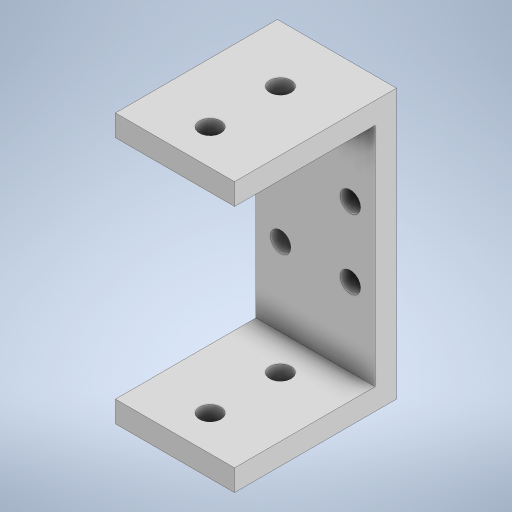
# Autodesk Inventor part: AcopleActuadorCarro
Saved by Autodesk Inventor 2023 (Build 270158000, 158)
## iProperties
Created: 2023-04-08
Part Number: AcopleActuadorCarro
Material: Generic
Document SubType Name: Modeling
Designer: Lenovo
Density: 1 g/cm^3
Appearance: Default
Author: Lenovo
Autodesk Inventor part; units mm, degrees
ref_plane "YZ Plane" through (0, 0, 0) normal (1, 0, 0) x (0, 1, 0)
ref_plane "XZ Plane" through (0, 0, 0) normal (0, 1, 0) x (-1, 0, 0)
ref_plane "XY Plane" through (0, 0, 0) normal (0, 0, 1) x (1, 0, 0)
sketch "Sketch1" plane through (0, 0, 0) normal (0, 0, 1) x (1, 0, 0)
  line L0 (-6, 110.6647) -> (-6, 110.2647)
  arc A0 (-6, 110.2647) -> (-5.6, 109.8647) centre (-5.6, 110.2647) ccw
  line L1 (-5.6, 109.8647) -> (-4.9, 109.8647)
  arc A1 (-4.9, 109.8647) -> (-4.7, 110.0647) centre (-4.9, 110.0647) ccw
  line L2 (-4.7, 110.0647) -> (-4.7, 110.3147)
  arc A2 (-4.5, 110.5147) -> (-4.7, 110.3147) centre (-4.5, 110.3147) ccw
  line L3 (-4.5, 110.5147) -> (-1.8, 110.5147)
  arc A3 (-1.4, 110.1147) -> (-1.8, 110.5147) centre (-1.8, 110.1147) ccw
  line L4 (-1.4, 110.1147) -> (-1.4, 104.4147)
  line L5 (-1.8, 104.0147) -> (-4.5, 104.0147)
  arc A4 (-1.8, 104.0147) -> (-1.4, 104.4147) centre (-1.8, 104.4147) ccw
  arc A5 (-4.7, 104.2147) -> (-4.5, 104.0147) centre (-4.5, 104.2147) ccw
  line L6 (-4.7, 104.2147) -> (-4.7, 104.4647)
  arc A6 (-4.7, 104.4647) -> (-4.9, 104.6647) centre (-4.9, 104.4647) ccw
  line L7 (-4.9, 104.6647) -> (-5.6, 104.6647)
  arc A7 (-5.6, 104.6647) -> (-6, 104.2647) centre (-5.6, 104.2647) ccw
  line L8 (-6, 104.2647) -> (-6, 103.6647)
  line L9 (-6.5, 116.6647) -> (-6.5, 110.6647)
  line L10 (-6.5, 110.6647) -> (-2.5, 110.6647)
  line L11 (-1.05, 103.6647) -> (-6.5, 103.6647)
  line L12 (-6.5, 103.6647) -> (-6.5, 97.1647)
  line L13 (-6.5, 97.1647) -> (-1.05, 97.1647)
  line L14 (-6, 97.1647) -> (-6, 96.5647)
  arc A8 (-6, 96.5647) -> (-5.6, 96.1647) centre (-5.6, 96.5647) ccw
  line L15 (-5.6, 96.1647) -> (-4.9, 96.1647)
  arc A9 (-4.9, 96.1647) -> (-4.7, 96.3647) centre (-4.9, 96.3647) ccw
  arc A10 (-4.5, 96.8147) -> (-4.7, 96.6147) centre (-4.5, 96.6147) ccw
  line L16 (-4.7, 96.3647) -> (-4.7, 96.6147)
  line L17 (-4.5, 96.8147) -> (-1.8, 96.8147)
  arc A11 (-1.4, 96.4147) -> (-1.8, 96.8147) centre (-1.8, 96.4147) ccw
  line L18 (-1.4, 96.4147) -> (-1.4, 90.7147)
  arc A12 (-1.8, 90.3147) -> (-1.4, 90.7147) centre (-1.8, 90.7147) ccw
  line L19 (-1.8, 90.3147) -> (-4.5, 90.3147)
  arc A13 (-4.7, 90.5147) -> (-4.5, 90.3147) centre (-4.5, 90.5147) ccw
  line L20 (-4.7, 90.5147) -> (-4.7, 90.7647)
  arc A14 (-4.7, 90.7647) -> (-4.9, 90.9647) centre (-4.9, 90.7647) ccw
  line L21 (-4.9, 90.9647) -> (-5.6, 90.9647)
  arc A15 (-5.6, 90.9647) -> (-6, 90.5647) centre (-5.6, 90.5647) ccw
  line L22 (-6, 90.5647) -> (-6, 90.1647)
  line L23 (-2.5, 90.1647) -> (-6.5, 90.1647)
  line L24 (-6.5, 90.1647) -> (-6.5, 84.1647)
  line L25 (32.5, 123.1647) -> (0, 123.1647)
  circle A16 centre (0, 116.6647) radius 4.75
  circle A17 centre (32.5, 116.6647) radius 4.75
  circle A18 centre (0, 84.1647) radius 4.75
  circle A19 centre (32.5, 84.1647) radius 4.75
  line L26 (39, 97.1647) -> (39, 103.6647)
  line L27 (39, 110.6647) -> (39, 116.6647)
  line L28 (39, 84.1647) -> (39, 90.1647)
  line L29 (26.5, 77.6647) -> (32.5, 77.6647)
  line L30 (0, 77.6647) -> (6, 77.6647)
  line L31 (13, 77.6647) -> (19.5, 77.6647)
  circle A20 centre (16.25, 100.4147) radius 15
  circle A21 centre (16.2588, 5.0016) radius 2.5
  circle A22 centre (16.25, -50.5) radius 2.5
  circle A23 centre (16.25, 100.4147) radius 5
  circle A24 centre (16.25, 100.4147) radius 8.45
  line L32 (24.75, 95.5072) -> (24.75, 105.3221)
  line L33 (44, 10) -> (-11.5, 10)
  line L34 (-11.5, 10) -> (-11.5, -55.5)
  line L35 (-11.5, -55.5) -> (44, -55.5)
  line L36 (44, -55.5) -> (44, 10)
  line L37 (-11.5, 30) -> (44, 30)
  line L38 (-11.5, -75.5) -> (-11.5, 30)
  line L39 (44, 30) -> (44, -75.5)
  line L40 (44, -75.5) -> (-11.5, -75.5)
  circle A25 centre (16.25, -65.5) radius 5
  circle A26 centre (16.25, 20) radius 5
  line L41 (-11.5, 37.6647) -> (44, 37.6647)
  line L42 (44, 37.6647) -> (44, 163.1647)
  line L43 (44, 163.1647) -> (-11.5, 163.1647)
  line L44 (-11.5, 163.1647) -> (-11.5, 37.6647)
  line L45 (-11.5, 163.1647) -> (44, 37.6647)
  line L46 (16.25, 100.4147) -> (112.1111, 100.4147)
  dimension "d2" = 125.5
  constraints: 94 end point, 32 point on circle, 27 centre point, 2 horizontal, 2 parallel, 1 midpoint, 1 perpendicular
  measures "d2" distance of L42.end L41.end
extrude "Extrusion1" add sketch "Sketch1" along normal blind 10 contours L46 A24 L45 A20 | L46 L42 L45 A20 | A20 L45 A24 L46 | A20 L45 L43 L42 L46 | L45 A24 A20 | A20 L45 L41 L44 | L45 A23 A24 | A24 L46 A23 L45 | L45 A23 L46 A24 | L45 A23 | A23 L46 L45 | L45 L46 A23
sketch "Sketch2" plane through (0, 0, 10) normal (0, 0, 1) x (1, 0, 0)
  line L0 (44, 163.1647) -> (-11.5, 163.1647) projected
  line L1 (44, 37.6647) -> (44, 163.1647) projected
  line L2 (-11.5, 163.1647) -> (44, 163.1647)
  line L3 (44, 163.1647) -> (44, 153.1647)
  line L4 (44, 153.1647) -> (-11.5, 153.1647)
  line L5 (-11.5, 153.1647) -> (-11.5, 163.1647)
  line L6 (-11.5, 37.6647) -> (44, 37.6647)
  line L7 (44, 37.6647) -> (44, 47.6647)
  line L8 (44, 47.6647) -> (-11.5, 47.6647)
  line L9 (-11.5, 47.6647) -> (-11.5, 37.6647)
  point P0 (0, 0)
  dimension "d5" = 10
  dimension "d6" = 10
  constraints: 16 end point, 4 parallel, 3 point on line, 2 horizontal, 2 perpendicular
  measures "d5" distance of L2.end L3.end
  measures "d6" distance of L7.end L6.end
extrude "Extrusion2" add sketch "Sketch2" along normal blind 65.5
sketch "Sketch3" plane through (-11.5, 163.1647, 0) normal (0, 1, 0) x (1, 0, 0)
  line L0 (0, -10) -> (55.5, -10) projected
  line L1 (0, -10) -> (0, -75.5) projected
  line L2 (55.5, -10) -> (0, -10)
  line L3 (0, -10) -> (0, -75.5)
  line L4 (0, -75.5) -> (55.5, -75.5)
  line L5 (55.5, -75.5) -> (55.5, -10)
  line L6 (55.5, -10) -> (55.5, -75.5) projected
  line L7 (55.5, -42.75) -> (0, -42.75)
  line L8 (55.5, -10) -> (0, -42.75)
  line L9 (27.75, -26.375) -> (27.75, -42.75)
  line L10 (55.5, -42.75) -> (0, -75.5)
  line L11 (27.75, -59.125) -> (27.75, -42.75)
  circle A0 centre (27.75, -26.375) radius 5
  circle A1 centre (27.75, -59.125) radius 5
  point P0 (11.5, 0)
  dimension "d9" = 10
  dimension "d10" = 10
  constraints: 18 end point, 5 midpoint, 4 equal length, 2 centre point, 2 coincident, 1 horizontal, 1 perpendicular
  measures "d9" diameter of A0
  measures "d10" diameter of A1
extrude "Extrusion3" cut sketch "Sketch3" against normal through all contours A0 L9 L8 | L8 A0 | L8 L9 A0 | A1 L10 | L10 L11 A1 | A1 L11 L10
body "Solid1"
